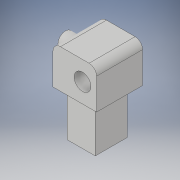
# Autodesk Inventor part: Shoulder1 Link-lrg
Saved by Autodesk Inventor 2017 (Build 210142000, 142)
## iProperties
Created: 2017-05-25
Part Number: Shoulder1 Link-lrg
Material: Generic
Document SubType Name: Modeling
Designer: garre
Density: 1 g/cm^3
Appearance: Default
Author: garre
Autodesk Inventor part; units mm, degrees
ref_plane "YZ Plane" through (0, 0, 0) normal (1, 0, 0) x (0, 1, 0)
ref_plane "XZ Plane" through (0, 0, 0) normal (0, 1, 0) x (-1, 0, 0)
ref_plane "XY Plane" through (0, 0, 0) normal (0, 0, 1) x (1, 0, 0)
sketch "Sketch1" plane through (0, 0, 0) normal (0, 0, 1) x (1, 0, 0)
  circle A0 centre (0, 0) radius 34.29
  line L0 (-120.65, -78.74) -> (120.65, -78.74)
  line L1 (120.65, -78.74) -> (120.65, 48.26)
  line L2 (90.17, 78.74) -> (-90.17, 78.74)
  line L3 (-120.65, 48.26) -> (-120.65, -78.74)
  arc A1 (-90.17, 78.74) -> (-120.65, 48.26) centre (-90.17, 48.26) ccw
  arc A2 (120.65, 48.26) -> (90.17, 78.74) centre (90.17, 48.26) ccw
  point P0 (120.65, 78.74)
  point P1 (-120.65, 78.74)
  dimension "d0" = 68.58
  dimension "d1" = 157.48
  dimension "d2" = 241.3
  dimension "d3" = 78.74
  dimension "d4" = 120.65
  dimension "d5" = 30.48
  constraints: 8 end point, 4 point on circle, 4 point on line, 4 tangent, 3 centre point, 2 parallel, 1 coincident, 1 equal radius, 1 horizontal, 1 perpendicular
  measures "d0" diameter of A0
  measures "d1" distance of L0.end point (120.65, 78.74)
  measures "d2" distance of point (120.65, 78.74) point (-120.65, 78.74)
  measures "d3" distance from line of L2 A0.centre
  measures "d4" distance from line of L1 point (0, 0)
  measures "d5" radius of A1
extrude "Extrusion1" add sketch "Sketch1" against normal blind 187.96
sketch "Sketch2" plane through (0, 0, -187.96) normal (0, 0, -1) x (-1, 0, 0)
  circle A0 centre (0, 0) radius 34.29 projected
  circle A1 centre (0, 0) radius 52.0012
  constraints: 1 centre point, 1 coincident
extrude "Extrusion2" add sketch "Sketch2" against normal blind 101.6 contours A0 | A1
sketch "Sketch3" plane through (-120.65, -78.74, 0) normal (-1, 0, 0) x (0, 0, 1)
  line L0 (-187.96, 0) -> (-187.96, 127) projected
  line L1 (-187.96, 127) -> (-58.42, 127)
  line L2 (-58.42, -30.48) -> (-58.42, -215.9)
  line L3 (-58.42, -215.9) -> (-187.96, -215.9)
  line L4 (-187.96, -215.9) -> (-187.96, 127)
  line L5 (0, 0) -> (-187.96, 0) projected
  line L6 (-27.94, 0) -> (0, 0)
  line L7 (-187.96, -215.9) -> (-58.42, -215.9)
  line L8 (-58.42, -215.9) -> (-58.42, -30.48)
  line L9 (-58.42, 0) -> (-187.96, 0)
  line L10 (-187.96, 0) -> (-187.96, -215.9)
  arc A0 (-27.94, 0) -> (-58.42, -30.48) centre (-27.94, -30.48) ccw
  line L11 (0, 0) -> (-187.96, 0)
  line L12 (-187.96, -215.9) -> (-58.42, -215.9)
  arc A1 (-27.94, 0) -> (-58.42, -30.48) centre (-27.94, -30.48) ccw
  line L13 (-58.42, -30.48) -> (-58.42, -215.9)
  line L14 (-187.96, -215.9) -> (-187.96, 0)
  line L15 (-187.96, 0) -> (-27.94, 0)
  arc A2 (-27.94, 0) -> (-58.42, -30.48) centre (-27.94, -30.48) ccw
  point P0 (0, 78.74)
  dimension "d10" = 129.54
  dimension "d11" = 342.9
  dimension "d12" = 30.48
  constraints: 28 end point, 6 point on circle, 4 collinear, 4 parallel, 4 point on line, 4 tangent, 3 centre point, 2 horizontal, 2 perpendicular, 1 coincident, 1 vertical
  measures "d10" distance of L2.end L3.end
  measures "d11" distance of L3.end L0.end
  measures "d12" radius of A0
extrude "Extrusion3" add sketch "Sketch3" against normal blind 114.3
fillet "Fillet1" radius 30.48 1 edges at (-6.35, -78.74, -107.95)
sketch "Sketch4" plane through (-120.65, -78.74, 0) normal (-1, 0, 0) x (0, 0, 1)
  line L0 (0, 127) -> (-187.96, 127) projected
  line L1 (-187.96, 127) -> (-187.96, 69.85)
  line L2 (-187.96, 127) -> (-187.96, 0) projected
  line L3 (-144.78, 78.74) -> (-114.3, 78.74)
  circle A0 centre (-114.3, 78.74) radius 30.48
  line L4 (0, 127) -> (0, 0) projected
  point P0 (0, 78.74)
  dimension "d18" = 60.96
  dimension "d17" = 57.15
  dimension "d21" = 114.3
  dimension "d25" = 0
  constraints: 4 end point, 1 coincident, 1 horizontal, 1 horizontal alignment, 1 point on line, 2 other
  measures "d17" distance of L0.end L1.end
  measures "d21" distance from line of L4 L3.end
  measures "d25" vertical distance of point (0, 78.74) L3.end
extrude "Extrusion4" add sketch "Sketch4" along normal blind 63.5
sketch "Sketch5" plane through (120.65, -78.74, 0) normal (1, 0, 0) x (0, 0, -1)
  line L0 (-23.8125, -17.4625) -> (228.6, -17.4625)
  line L1 (228.6, -17.4625) -> (228.6, 187.325)
  line L2 (228.6, 187.325) -> (-23.8125, 187.325)
  line L3 (-23.8125, 187.325) -> (-23.8125, -17.4625)
  point P0 (0, 78.74)
  constraints: 8 end point, 2 parallel, 1 horizontal, 1 perpendicular
extrude "Extrusion5" cut sketch "Sketch5" against normal blind 63.5
fillet "Fillet2" radius 30.48 1 edges at (57.15, 78.74, -93.98)
equation "\"d3\" = 0.5 * d1"
equation "\"d4\" = 0.5 * d2"
body "Solid1"
